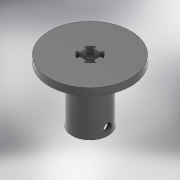
# Autodesk Inventor part: BearingInsert
Saved by Autodesk Inventor 2020.3 (Build 243373000, 373)
## iProperties
Created: 2021-08-03
Part Number: BearingInsert
Material: ABS Plastic
Document SubType Name: Modeling
Designer: justi
Density: 1.06 g/cm^3
Appearance: Smooth - Black
Author: justi
Autodesk Inventor part; units mm, degrees
ref_plane "XZ Plane" through (0, 0, 0) normal (0, 1, 0) x (-1, 0, 0)
ref_plane "XY Plane" through (0, 0, 0) normal (0, 0, 1) x (1, 0, 0)
sketch "Sketch1" plane through (0, 0, 0) normal (1, 0, 0) x (0, 1, 0)
  line L0 (0, 28.5) -> (5, 28.5)
  line L1 (5, 28.5) -> (5, 0)
  line L2 (5, 0) -> (0, 0)
  line L3 (0, 0) -> (-38, 0)
  line L4 (-38, 0) -> (-38, 12.5)
  line L5 (-38, 12.5) -> (0, 12.5)
  line L6 (0, 12.5) -> (0, 28.5)
  line L7 (-46.6, 0) -> (13.6, 0) projected
  dimension "d0" = 28.5
  dimension "d1" = 5
  dimension "d2" = 38
  dimension "d3" = 12.5
  constraints: 14 end point, 3 perpendicular, 2 horizontal, 1 vertical
  measures "d0" distance of L2.end L0.start
  measures "d1" distance of L0.start L0.end
  measures "d2" distance of L2.end L3.end
  measures "d3" distance of L3.end L4.end
revolve "Revolution1" add sketch "Sketch1" angle 360 about axis through (0, -10, 0) along (0, 1, 0)
sketch "Sketch2" plane through (0, -38, 0) normal (0, -1, 0) x (1, 0, 0)
  circle A0 centre (0, 0) radius 10
  dimension "d5" = 20
  constraints: 1 centre point, 1 coincident
  measures "d5" diameter of A0
extrude "Extrusion1" cut sketch "Sketch2" against normal blind 25
sketch "Sketch3" plane through (0, 5, 0) normal (0, 1, 0) x (1, 0, 0)
  point P0 (0, 0)
  point P1 (0, 0)
  constraints: 1 coincident
hole "Hole1" at (0, 5, 0) direction (0, -1, 0) diameter 6.6 end through all counterbore diameter 14.55 counterbore depth 5 clearance for "Hex Head Bolt" size "M6" standard "Ansi Metric M Profile"
sketch "Sketch5" plane through (0, 0, 0) normal (0, 1, 0) x (1, 0, 0)
  line L0 (-2.5, 9.775) -> (2.5, 9.775)
  line L1 (2.5, 9.775) -> (2.5, 4.775)
  line L2 (2.5, 4.775) -> (-2.5, 4.775)
  line L3 (-2.5, 4.775) -> (-2.5, 9.775)
  circle A0 centre (0, 0) radius 7.275 projected
  line L4 (-2.5, 9.775) -> (2.5, 4.775) construction
  line L5 (2.5, 9.775) -> (-2.5, 4.775) construction
  line L6 (-9.775, -2.5) -> (-4.775, -2.5)
  line L7 (-4.775, -2.5) -> (-4.775, 2.5)
  line L8 (-4.775, 2.5) -> (-9.775, 2.5)
  line L9 (-9.775, 2.5) -> (-9.775, -2.5)
  line L10 (-9.775, -2.5) -> (-4.775, 2.5) construction
  line L11 (-4.775, -2.5) -> (-9.775, 2.5) construction
  line L12 (-2.5, -9.775) -> (2.5, -9.775)
  line L13 (2.5, -9.775) -> (2.5, -4.775)
  line L14 (2.5, -4.775) -> (-2.5, -4.775)
  line L15 (-2.5, -4.775) -> (-2.5, -9.775)
  line L16 (-2.5, -9.775) -> (2.5, -4.775) construction
  line L17 (2.5, -9.775) -> (-2.5, -4.775) construction
  line L18 (4.775, -2.5) -> (9.775, -2.5)
  line L19 (9.775, -2.5) -> (9.775, 2.5)
  line L20 (9.775, 2.5) -> (4.775, 2.5)
  line L21 (4.775, 2.5) -> (4.775, -2.5)
  line L22 (4.775, -2.5) -> (9.775, 2.5) construction
  line L23 (9.775, -2.5) -> (4.775, 2.5) construction
  point P0 (0, 7.275)
  point P1 (-7.275, 0)
  point P2 (0, -7.275)
  point P3 (7.275, 0)
  point P4 (-2.5, -6.832)
  point P5 (2.5, -6.832)
  point P6 (-6.832, 2.5)
  point P7 (-6.832, -2.5)
  point P8 (2.5, 6.832)
  point P9 (-2.5, 6.832)
  point P10 (6.832, -2.5)
  point P11 (6.832, 2.5)
  dimension "d19" = 5
  dimension "d20" = 5
  dimension "d21" = 5
  dimension "d22" = 5
  dimension "d23" = 5
  dimension "d24" = 5
  dimension "d25" = 5
  dimension "d26" = 5
  constraints: 48 end point, 8 midpoint, 8 parallel, 4 horizontal, 4 perpendicular, 4 point on line, 2 other
  measures "d19" distance of L1.end L2.end
  measures "d20" distance of L0.end L1.end
  measures "d21" distance of L8.end L7.end
  measures "d22" distance of L7.end L6.end
  measures "d23" distance of L14.end L13.end
  measures "d24" distance of L13.end L12.end
  measures "d25" distance of L20.end L19.end
  measures "d26" distance of L19.end L18.end
extrude "Extrusion3" add sketch "Sketch5" along normal up to surface (5 mm away) contours A0 L1 L2 L3 | L8 L7 L6 A0 | A0 L18 L21 L20 | L15 L14 L13 A0
ref_plane "Work Plane1" through (12.5, 0, 0) normal (1, 0, 0) x (0, 1, 0)
sketch "Sketch7" plane through (12.5, 0, 0) normal (1, 0, 0) x (0, 1, 0)
  line L0 (-38, -10) -> (-38, 10) projected
  line L1 (-38, 0) -> (-33, 0)
  point P0 (0, 0)
  dimension "d38" = 5
  constraints: 2 end point, 1 horizontal, 1 midpoint
  measures "d38" distance of L1.start L1.end
hole "Hole3" at (12.5, -33, 0) direction (-1, 0, 0) diameter 5.5 end through all clearance for "Hex Head Bolt" size "M5" standard "Ansi Metric M Profile"
body "Solid1"
